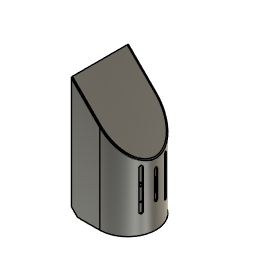
SimpleLampshade (Autodesk Fusion 360 design; units mm, degrees)
Autodesk Fusion 360 part; units mm, degrees
sketch "Sketch1" plane through (0, 0, 0) normal (0, 0, 1) x (1, 0, 0) in component "Lampshade"
  circle A0 centre (0, 0) radius 23.5
  circle A1 centre (0, 0) radius 25.1
  circle A2 centre (0, -23.5) radius 5
  line L0 (0, 0) -> (0, -25.1) construction
  circle A3 centre (0, -23.5) radius 4
  line L1 (0, -23.5) -> (-4.3301, -26)
  circle A4 centre (0, 0) radius 45.1
  circle A5 centre (0, 0) radius 46.7
  line L2 (-0.8, -23.4864) -> (0.8, -23.4864)
  line L3 (0.8, -23.4864) -> (0.8, -46.6931)
  line L4 (0.8, -46.6931) -> (-0.8, -46.6931)
  line L5 (-0.8, -46.6931) -> (-0.8, -23.4864)
  line L6 (-0.8, -46.6931) -> (-0.8, 46.6931)
  dimension "d1" = 47
  dimension "d3" = 1.6
  dimension "d4" = 10
  dimension "d5" = 1
  dimension "d6" = 120
  dimension "d18" = 20
  dimension "d19" = 1.6
  dimension "d20" = 1.6
  constraint coincident A0.centre A1.centre
  constraint concentric A0 A1
  constraint coincident A0 A2.centre
  constraint vertical L0
  constraint coincident A2.centre L0
  constraint concentric A2 A3
  constraint coincident A2.centre A3.centre
  constraint coincident A1 L0.end
  constraint coincident A2 L1.end
  constraint horizontal L2
  constraint vertical L3
  constraint horizontal L4
  constraint vertical L5
  constraint coincident A0 L2.start
  constraint coincident A0 L2.end
  constraint coincident A5 L3.end
  constraint coincident A5 L6.end
  constraint perpendicular L4 L6
  measures "d1" diameter of A0
  measures "d3" distance of A0 A1
  measures "d4" diameter of A2
  measures "d5" distance of A2 A3
  measures "d6" angle of L0 L1
  measures "d18" distance of A1 A4
  measures "d19" distance of A4 A5
  measures "d20" distance of L3 L5
extrude "Extrude1" add sketch "Sketch1" along normal blind 30 contours A0 A1 A3 L1 L5 L6 | A0 L1 L5 L6 | A0 A1 L1 L3 L5 L6 | A0 A1 A2 A3 | A0 A1 A3 L3 | A1 L1 L5 L6 | A0 A1 A2 L6 | A0 A1 A2 A3 | A0 A1 A2 L6 makes body 1 in component "Lampshade"
extrude "Extrude2" add sketch "Sketch1" along normal up to surface (30 mm away) separate body contours A0 A2 A3 L6 | A0 A2 A3 L6 makes body 2 in component "Lampshade"
extrude "Extrude3" add sketch "Sketch1" along normal blind 20 separate body contours A0 L2 | A0 A3 L2 L6 | A0 A3 L6 | A0 A2 A3 L6 | A0 A2 A3 L6 | A0 A2 L6 | A0 A2 L6 makes body 3 in component "Lampshade"
chamfer "Chamfer1" distance 20 angle 45 1 edges at (-21.9097, -8.498, 20) 1 faces at (-8.9233, 1.6941, 20) on bodies 3 in component "Lampshade"
combine "Combine2" operation cut target body 2 tool bodies 3 in component "Lampshade"
pattern_circular "C-Pattern2" count 6 over 360 about axis through (0, 0, 1.75) along (0, 0, 1) of bodies 2 makes body 4 at (20.9209, -6.7825, 11.02) makes body 5 at (16.3343, 14.7268, 11.02) makes body 6 at (-4.5866, 21.5093, 11.02) makes body 7 at (-20.9209, 6.7825, 11.02) makes body 8 at (-16.3343, -14.7268, 11.02) in component "Lampshade"
extrude "Extrude4" add sketch "Sketch1" along normal up to surface (30 mm away) separate body contours A1 A3 L3 L5 L6 | A2 A3 L3 L5 L6 | A2 A4 L3 L5 L6 makes body 9 in component "Lampshade"
extrude "Extrude5" add sketch "Sketch1" along normal blind 195 separate body contours A4 A5 L3 L6 | A4 L3 L4 L5 L6 makes body 10 in component "Lampshade"
pattern_circular "C-Pattern3" count 5 over 180 about axis through (0, 0, 1.75) along (0, 0, 1) of bodies 9 makes body 11 at (24.5988, -23.4675, 20) makes body 12 at (33.988, 0.8, 10) makes body 13 at (23.4675, 24.5988, 20) makes body 14 at (-0.8, 33.988, 10) in component "Lampshade"
extrude "Extrude6" add 2 faces at (-0.8, 45.6263, 65) (-0.8, -46.1597, 65) along direction (-1, 0, 0) blind 45 on bodies 10 bodies 9 10 14 in component "Lampshade"
ref_plane "WorkPlane2" through (-45.8, 45.893, 195) normal (0.707107, 0, 0.707107) x (0, 1, 0)
split "Split1" by plane through (-45.8, 45.893, 195) normal (0.707107, 0, 0.707107) bodies 9 makes body 15 at (6.2031, -46.2862, 160.8667) in component "Lampshade"
delete_body "RemoveBody1" bodies 15 in component "Lampshade"
sketch "Sketch2" plane through (74.6, 0, 74.6) normal (0.707107, 0, 0.707107) x (0, 1, 0) in component "Lampshade"
  line L0 (45.0929, 170.2713) -> (45.0929, 106.6317)
  ellipse E0 centre (0, 105.5003) end of major axis (0, 41.7193) minor radius 45.1 (-45.0929, 106.6317) -> (45.0929, 106.6317) ccw
  line L1 (-45.0929, 106.6317) -> (-45.0929, 170.2713)
  line L2 (-45.0929, 170.2713) -> (-46.6931, 170.2713)
  line L3 (-46.6931, 170.2713) -> (-46.6931, 104.369)
  ellipse E1 centre (0, 105.5003) end of major axis (0, 39.4566) minor radius 46.7 (-46.6931, 104.369) -> (46.6931, 106.6317) ccw
  line L4 (46.6931, 106.6317) -> (46.6931, 170.2713)
  line L5 (46.6931, 170.2713) -> (45.0929, 170.2713)
  line L6 (46.6931, 170.2713) -> (-46.6931, 170.2713)
  constraint coincident L4.end L5.start
  constraint coincident L2.end L3.start
extrude "Extrude8" add sketch "Sketch2" against normal blind 1.6 separate body makes body 16 in component "Lampshade"
sketch "Sketch3" plane through (0, 46.6931, 0) normal (0, 1, 0) x (-1, 0, 0) in component "Lampshade"
  line L0 (0.8, 150) -> (0.8, 0)
  line L1 (0.8, 0) -> (45.8, 0)
  line L2 (46.9314, 193.8686) -> (1.9314, 148.8686)
  line L3 (45.8, 195) -> (46.9314, 193.8686)
  line L4 (45.8, 195) -> (45.8, 0)
  line L5 (45.8, 195) -> (45.8, 192.7373)
  line L6 (45.8, 192.7373) -> (46.9314, 193.8686)
  line L7 (46.9314, 193.8686) -> (45.8, 195)
  constraint coincident L3.start L4.start
  constraint coincident L2 L5.end
  constraint coincident L4 L5.end
  constraint coincident L2.start L3.end
extrude "Extrude9" cut sketch "Sketch3" against normal through all bodies 16 in component "Lampshade"
sketch "Sketch4" plane through (0, 0, 0) normal (1, 0, 0) x (0, 1, 0) in component "Lampshade"
  line L0 (0, 0) -> (0, 65) construction
  line L1 (-2.5, 40) -> (2.5, 40)
  line L2 (2.5, 40) -> (2.5, 90)
  line L3 (2.5, 90) -> (-2.5, 90)
  line L4 (-2.5, 90) -> (-2.5, 40)
  line L5 (-2.5, 40) -> (2.5, 90) construction
  line L6 (2.5, 40) -> (-2.5, 90) construction
  line L7 (-50, 65) -> (50, 65) construction
  line L8 (-17.5, 100) -> (-22.5, 100)
  line L9 (-22.5, 100) -> (-22.5, 30)
  line L10 (-22.5, 30) -> (-17.5, 30)
  line L11 (-17.5, 30) -> (-17.5, 100)
  line L12 (-17.5, 100) -> (-22.5, 30) construction
  line L13 (-22.5, 100) -> (-17.5, 30) construction
  line L14 (22.5, 100) -> (17.5, 100)
  line L15 (17.5, 100) -> (17.5, 30)
  line L16 (17.5, 30) -> (22.5, 30)
  line L17 (22.5, 30) -> (22.5, 100)
  line L18 (22.5, 100) -> (17.5, 30) construction
  line L19 (17.5, 100) -> (22.5, 30) construction
  line L20 (20, 100) -> (22.5, 97.5)
  line L21 (20, 100) -> (23.5355, 100) construction
  line L22 (20, 100) -> (17.5, 97.5)
  line L23 (20, 30) -> (22.5, 32.5)
  line L24 (0, 40) -> (-2.5, 42.5)
  line L25 (0, 40) -> (2.5, 42.5)
  line L26 (0, 90) -> (2.5, 87.5)
  line L27 (0, 90) -> (-2.5, 87.5)
  line L28 (-20, 100) -> (-17.5, 97.5)
  line L29 (-20, 100) -> (-22.5, 97.5)
  line L30 (-20, 30) -> (-22.5, 32.5)
  line L31 (-20, 30) -> (-17.5, 32.5)
  line L32 (20, 30) -> (17.5, 32.5)
  line L33 (20, 30) -> (23.5355, 30) construction
  point P0 (0, 65)
  point P1 (-20, 65)
  point P2 (20, 65)
  dimension "d36" = 65
  dimension "d37" = 5
  dimension "d38" = 50
  dimension "d39" = 100
  dimension "d40" = 5
  dimension "d41" = 70
  dimension "d42" = 20
  dimension "d43" = 5
  dimension "d44" = 70
  dimension "d45" = 20
  dimension "d47" = 45
  dimension "d48" = 135
  constraint coincident L0.start origin
  constraint vertical L0
  constraint horizontal L1
  constraint perpendicular L1 L2
  constraint parallel L1 L3
  constraint parallel L2 L4
  constraint coincident L5 P0
  constraint coincident L6 P0
  constraint coincident P0 L0.end
  constraint perpendicular L2 L7
  constraint horizontal L8
  constraint perpendicular L8 L9
  constraint parallel L8 L10
  constraint parallel L9 L11
  constraint coincident L12 P1
  constraint coincident L13 P1
  constraint coincident L7 P1
  constraint midpoint P0 L7
  constraint horizontal L14
  constraint perpendicular L14 L15
  constraint parallel L14 L16
  constraint parallel L15 L17
  constraint coincident L18 P2
  constraint coincident L19 P2
  constraint coincident L7 P2
  constraint horizontal L21
  constraint midpoint L14 L20.start
  constraint coincident L17 L20.end
  constraint perpendicular L20 L22
  constraint midpoint L16 L23.start
  constraint coincident L17 L23.end
  constraint midpoint L1 L24.start
  constraint coincident L4 L24.end
  constraint perpendicular L23 L24
  constraint coincident L2 L25.end
  constraint perpendicular L24 L25
  constraint midpoint L3 L26.start
  constraint coincident L2 L26.end
  constraint perpendicular L25 L26
  constraint perpendicular L26 L27
  constraint midpoint L8 L28.start
  constraint coincident L11 L28.end
  constraint perpendicular L27 L28
  constraint perpendicular L28 L29
  constraint midpoint L10 L30.start
  constraint perpendicular L29 L30
  constraint perpendicular L30 L31
  constraint horizontal L33
  constraint coincident L15 L32.end
  constraint perpendicular L23 L32
  constraint coincident L15 L22.end
  constraint coincident L4 L27.end
  constraint coincident L9 L30.end
  constraint coincident L11 L31.end
  constraint coincident L9 L29.end
  measures "d36" distance of L0.start P0
  measures "d37" distance of L2.end L3.end
  measures "d38" distance of L1.end L2.end
  measures "d39" distance of L7.start L7.end
  measures "d40" distance of L9.end L10.end
  measures "d41" distance of L8.end L9.end
  measures "d42" distance of P0 P1
  measures "d43" distance of L15.end L16.end
  measures "d44" distance of L14.end L15.end
  measures "d45" distance of P0 P2
  measures "d47" angle of L20 L21
  measures "d48" angle of L32 L33
extrude "Extrude10" cut sketch "Sketch4" along normal through all contours L2 L4 L24 L25 L26 L27 | L9 L11 L28 L29 L30 L31 | L15 L17 L20 L22 L23 L32 bodies 9 in component "Lampshade"
chamfer "Chamfer2" distance 10 angle 45 2 edges at (-45.8, -45.893, 0) (-45.8, 45.893, 0) on bodies 9 in component "Lampshade"
component "Lampshade" placed x (1, 0, 0) y (0, 1, 0) z (0, 0, 1) at (0, 0, 0)
